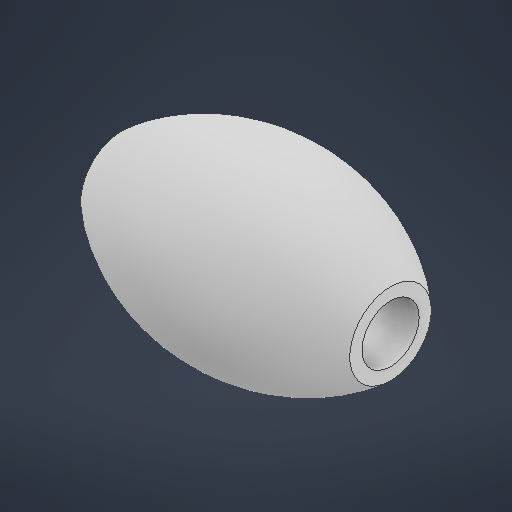
# Autodesk Inventor part: Part4
Saved by Autodesk Inventor 2026 (Build 300175000, 175)
## iProperties
Created: 2025-10-16
Part Number: Part4
Material: 一般
Document SubType Name: Modeling
Designer: masak
Density: 1 g/cm^3
Appearance: 既定
Author: masak
Autodesk Inventor part; units mm, degrees
ref_plane "YZ Plane" through (0, 0, 0) normal (1, 0, 0) x (0, 1, 0)
ref_plane "XZ Plane" through (0, 0, 0) normal (0, 1, 0) x (-1, 0, 0)
ref_plane "XY Plane" through (0, 0, 0) normal (0, 0, 1) x (1, 0, 0)
sketch "スケッチ1" plane through (0, 0, 0) normal (0, 1, 0) x (-1, 0, 0)
  line L0 (0, 0) -> (0, -3.5)
  line L1 (0, 0) -> (33, 0)
  line L2 (33, 0) -> (33, -3.5)
  line L3 (33, -3.5) -> (0, -3.5)
  line L4 (0, -3.5) -> (0, -5)
  line L5 (33, -3.5) -> (33, -5)
  arc A0 (0, -5) -> (33, -5) centre (16.5, 14.2526) ccw
  line L6 (0, 0) -> (0, -12)
  dimension "d0" = 3.5
  dimension "d1" = 33
  dimension "d2" = 1.5
  dimension "d4" = 12
  dimension "d5" = 1.5
  constraints: 14 end point, 5 vertical, 2 point on circle, 1 centre point, 1 horizontal, 1 perpendicular
  measures "d0" distance of L0.start L0.end
  measures "d1" distance of L0.start L1.end
  measures "d2" distance of L0.end L4.end
  measures "d4" distance of L0.start L6.end
  measures "d5" distance of L2.end L5.end
revolve "回転1" add sketch "スケッチ1" angle 360 about axis through (0, 0, 0) along (-1, 0, 0) contours L3 L5 A0 L4
